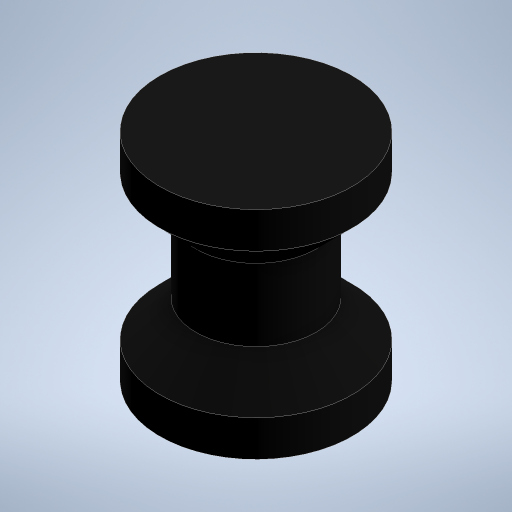
# Autodesk Inventor part: kolo_napedowe
Saved by Autodesk Inventor 2024.2 (Build 282272000, 272)
## iProperties
Created: 2024-01-12
Part Number: kolo_napedowe
Material: PLA
Document SubType Name: Modeling
Designer: Konrad
Density: 1 g/cm^3
Appearance: PLA
Author: Konrad
Autodesk Inventor part; units mm, degrees
ref_plane "YZ Plane" through (0, 0, 0) normal (1, 0, 0) x (0, 1, 0)
ref_plane "XZ Plane" through (0, 0, 0) normal (0, 1, 0) x (-1, 0, 0)
ref_plane "XY Plane" through (0, 0, 0) normal (0, 0, 1) x (1, 0, 0)
sketch "Szkic1" plane through (0, 0, 0) normal (0, 1, 0) x (-1, 0, 0)
  circle A0 centre (0, 0) radius 8
  circle A1 centre (0, 0) radius 5
  arc A2 (0.8292, 1.25) -> (0.8292, -1.25) centre (0, 0) ccw
  line L0 (0.8292, 1.25) -> (0.8292, -1.25)
  dimension "d2" = 1.5
  dimension "d3" = 2.5
  dimension "d4" = 10
  dimension "d5" = 16
  constraints: 3 centre point, 3 coincident, 2 end point, 2 point on circle, 1 vertical
  measures "d2" radius of A2
  measures "d3" distance of L0.start L0.end
  measures "d4" diameter of A1
  measures "d5" diameter of A0
extrude "Wyciągnięcie proste1" add sketch "Szkic1" along normal blind 18 contours A0 | A1 | L0 A2
extrude "Wyciągnięcie proste2" cut sketch "Szkic1" along normal blind 15 contours A0
extrude "Wyciągnięcie proste3" add sketch "Szkic1" along normal blind 3 contours A0
extrude "Wyciągnięcie proste4" cut sketch "Szkic1" along normal blind 8 contours L0 A2
chamfer "Faza1" distance 3 angle 45 2 edges at (5, 3, 0) (5, 15, 0)
